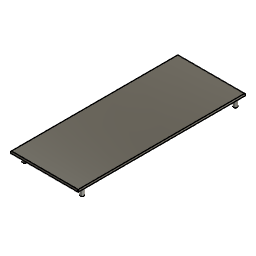
Top Plate v5 (Autodesk Fusion 360 design; units mm, degrees)
Autodesk Fusion 360 part; units mm, degrees
sketch "Sketch1" plane through (0, 0, 0) normal (0, 0, 1) x (1, 0, 0)
  line L0 (0, 0) -> (75, 0)
  line L1 (75, 0) -> (75, 200)
  line L2 (75, 200) -> (0, 200)
  line L3 (0, 200) -> (0, 0)
  circle A0 centre (0, 0) radius 2.5
  circle A1 centre (75, 0) radius 2.5
  circle A2 centre (75, 200) radius 2.5
  circle A3 centre (0, 200) radius 2.5
  line L4 (82.5, -20) -> (-7.5, -20)
  line L5 (-7.5, -20) -> (-7.5, 220)
  line L6 (-7.5, 220) -> (82.5, 220)
  line L7 (82.5, 220) -> (82.5, -20)
  line L8 (82.5, -20) -> (-7.5, 220) construction
  line L9 (-7.5, -20) -> (82.5, 220) construction
  point P0 (37.5, 100)
  dimension "d1" = 75
  dimension "d2" = 200
  dimension "d3" = 5
  dimension "d4" = 5
  dimension "d5" = 5
  dimension "d6" = 5
  dimension "d15" = 20
  dimension "d16" = 7.5
  constraint horizontal L0
  constraint vertical L1
  constraint horizontal L2
  constraint vertical L3
  constraint coincident L0.start L3.end
  constraint coincident L0.end L1.start
  constraint coincident L1.end L2.start
  constraint coincident L2.end L3.start
  constraint horizontal L4
  constraint perpendicular L4 L5
  constraint parallel L4 L6
  constraint parallel L5 L7
  constraint coincident L8 P0
  constraint coincident L9 P0
  measures "d1" distance of L0.start L0.end
  measures "d2" distance of L0.start L2.end
  measures "d3" diameter of A0
  measures "d4" diameter of A1
  measures "d5" diameter of A2
  measures "d6" diameter of A3
  measures "d15" distance of L2 L6
  measures "d16" distance of L3 L5
extrude "Extrude1" add sketch "Sketch1" against normal blind 5 contours L0 L3 A0 | L0 L3 A0 | L0 L1 A1 | L0 L1 A1 | L2 L3 A3 | L2 L3 A3 | L1 L2 A2 | L1 L2 A2 makes body 1 at (2.3492, 200.8551, -3.3333) makes body 2 at (2.4969, -0.1246, -3.3333) makes body 3 at (72.6508, 200.8551, -3.3333) makes body 4 at (77.4969, -0.1246, -3.3333)
sketch "Sketch2" plane through (0, 0, 0) normal (0, 0, 1) x (1, 0, 0)
  line L0 (80, -10) -> (-10, -10)
  line L1 (-10, -10) -> (-10, 210)
  line L2 (-10, 210) -> (80, 210)
  line L3 (80, 210) -> (80, -10)
  line L4 (80, -10) -> (-10, 210) construction
  line L5 (-10, -10) -> (80, 210) construction
  point P0 (35, 100)
  dimension "d13" = 220
  dimension "d14" = 90
  constraint horizontal L0
  constraint perpendicular L0 L1
  constraint parallel L0 L2
  constraint parallel L1 L3
  constraint coincident L4 P0
  constraint coincident L5 P0
  measures "d13" distance of L0.end L1.end
  measures "d14" distance of L1.end L2.end
extrude "Extrude2" add sketch "Sketch2" along normal blind 3 bodies 1 2 3 4
extrude "Extrude3" add 4 faces at (-0.8863, 0.2321, -5) (75.3045, -0.7757, -5) (74.3115, 199.2822, -5) (-0.6885, 199.2822, -5) along direction (0, 0, -1) blind 5 on bodies 1 bodies 1
chamfer "Chamfer1" distance 1 angle 45 4 faces at (-0.8863, 0.2321, -10) (75.3045, -0.7757, -10) (-0.6885, 199.2822, -10) (74.3115, 199.2822, -10) on bodies 1
chamfer "Chamfer2" distance 1.5 angle 45 4 faces at (80, 136.6667, 1) (50, -10, 1) (-10, 63.3333, 1) (20, 210, 1) on bodies 1
